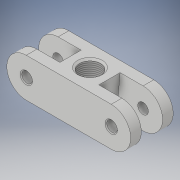
# Autodesk Inventor part: Součást25
Saved by Autodesk Inventor 2019 (Build 230136000, 136)
## iProperties
Created: 2020-01-28
Part Number: Součást25
Material: Všeobecné
Document SubType Name: Modeling
Designer: hynek
Density: 1 g/cm^3
Appearance: Výchozí
Author: hynek
Autodesk Inventor part; units mm, degrees
ref_plane "YZ Plane" through (0, 0, 0) normal (1, 0, 0) x (0, 1, 0)
ref_plane "XZ Plane" through (0, 0, 0) normal (0, 1, 0) x (-1, 0, 0)
sketch "Náčrt1" plane through (0, 0, 0) normal (0, 0, 1) x (1, 0, 0)
  line L0 (0, -15.4) -> (0, 15.4) construction
  line L1 (-49, 0) -> (49, 0) construction
  arc A0 (-24, 11) -> (-24, -11) centre (-24, 0) ccw
  arc A1 (24, -11) -> (24, 11) centre (24, 0) ccw
  line L2 (-24, 11) -> (24, 11)
  line L3 (-24, -11) -> (24, -11)
  circle A2 centre (-24, 0) radius 3
  circle A3 centre (24, 0) radius 3
  point P0 (0, 0)
  point P1 (0, -11)
  point P2 (0, 11)
  dimension "d0" = 22
  dimension "d1" = 22
  dimension "d2" = 48
  dimension "d3" = 6
  dimension "d4" = 6
  constraints: 4 centre point, 4 end point, 4 point on circle, 4 tangent, 3 point on line, 2 coincident, 2 midpoint
  measures "d0" diameter of A1
  measures "d1" diameter of A0
  measures "d2" distance of A1.centre A0.centre
  measures "d3" diameter of A2
  measures "d4" diameter of A3
extrude "Vysunutí1" add sketch "Náčrt1" along normal mid plane 24
ref_plane "Pracovní rovina1" through (0, 0, 6) normal (0, 0, 1) x (1, 0, 0)
sketch "Náčrt2" plane through (0, 0, 6) normal (0, 0, 1) x (1, 0, 0)
  line L0 (-56, 0) -> (56, 0) construction
  line L1 (0, -15.4) -> (0, 15.4) construction
  line L2 (11, 11) -> (9, -11)
  line L3 (9, -11) -> (40, -11)
  line L4 (40, -11) -> (40, 11)
  line L5 (40, 11) -> (11, 11)
  line L6 (24, 11) -> (-24, 11) construction
  line L7 (-24, -11) -> (24, -11) construction
  line L8 (-11, 11) -> (-9, -11)
  line L9 (-9, -11) -> (-40, -11)
  line L10 (-40, -11) -> (-40, 11)
  line L11 (-40, 11) -> (-11, 11)
  point P0 (0, 0)
  dimension "d10" = 11
  dimension "d11" = 9
  dimension "d12" = 40
  dimension "d15" = 0
  dimension "d16" = 0
  constraints: 16 end point, 4 symmetric about line, 2 perpendicular, 1 horizontal
  measures "d10" distance from line of L1 L2.start
  measures "d11" distance from line of L1 L2.end
  measures "d12" distance between parallel lines of L1 L4
  measures "d15" distance between parallel lines of L6 L5
  measures "d16" distance between parallel lines of L7 L3
extrude "Vysunutí3" cut sketch "Náčrt2" against normal blind 12
sketch "Náčrt3" plane through (-24, 11, -12) normal (0, 1, 0) x (1, 0, 0)
  circle A0 centre (24, -12) radius 6
  dimension "d19" = 12
  constraints: 1 centre point, 1 coincident
  measures "d19" diameter of A0
extrude "Vysunutí4" cut sketch "Náčrt3" against normal up to next
chamfer "Zkosení1" distance 1 angle 45 2 edges at (-6, 11, 0) (-6, -11, 0)
chamfer "Zkosení2" distance 0.5 angle 45 4 edges at (-27, 0, 12) (21, 0, 12) (21, 0, -12) (-27, 0, -12)
thread "Závit1" size "M12x1" class "6H" standard "ISO Metric profile" full length
